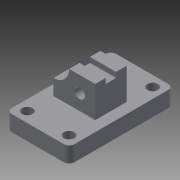
# Autodesk Inventor part: HW 8 Part6
Saved by Autodesk Inventor 2015 (Build 190159000, 159)
## iProperties
Created: 2016-03-08
Part Number: HW 8 Part6
Material: Generic
Document SubType Name: Modeling
Designer: Melissa
Density: 1 g/cm^3
Appearance: Default
Author: Melissa
Autodesk Inventor part; units mm, degrees
ref_plane "YZ Plane" through (0, 0, 0) normal (1, 0, 0) x (0, 1, 0)
ref_plane "XZ Plane" through (0, 0, 0) normal (0, 1, 0) x (-1, 0, 0)
ref_plane "XY Plane" through (0, 0, 0) normal (0, 0, 1) x (1, 0, 0)
sketch "Sketch1" plane through (0, 0, 0) normal (0, 0, 1) x (1, 0, 0)
  line L0 (0, 0) -> (50.8, 0)
  line L1 (50.8, 0) -> (50.8, 38.1)
  line L2 (50.8, 38.1) -> (19.05, 38.1)
  line L3 (0, 19.05) -> (0, 0)
  arc A0 (0, 19.05) -> (19.05, 38.1) centre (0, 38.1) ccw
  circle A1 centre (31.75, 19.05) radius 6.35
  dimension "d0" = 38.1
  dimension "d1" = 50.8
  dimension "d4" = 19.05
  dimension "d5" = 12.7
  dimension "d6" = 19.05
  dimension "d7" = 19.05
  constraints: 8 end point, 2 centre point, 2 horizontal, 2 perpendicular, 2 point on circle
  measures "d0" distance of L0.end L1.end
  measures "d1" distance of L0.start L0.end
  measures "d4" radius of A0
  measures "d5" diameter of A1
  measures "d6" distance from line of L1 A1.centre
  measures "d7" distance from line of L0 A1.centre
extrude "Extrusion1" add sketch "Sketch1" along normal blind 38.1
sketch "Sketch2" plane through (0, 0, 0) normal (0, -1, 0) x (1, 0, 0)
  line L0 (57.15, 82.55) -> (-6.35, 82.55)
  line L1 (-12.7, 76.2) -> (-12.7, -38.1)
  line L2 (-6.35, -44.45) -> (57.15, -44.45)
  line L3 (63.5, -38.1) -> (63.5, 76.2)
  line L4 (0, 0) -> (0, 38.1) projected
  line L5 (0, 0) -> (50.8, 0) projected
  arc A0 (63.5, 76.2) -> (57.15, 82.55) centre (57.15, 76.2) ccw
  arc A1 (-6.35, 82.55) -> (-12.7, 76.2) centre (-6.35, 76.2) ccw
  arc A2 (-12.7, -38.1) -> (-6.35, -44.45) centre (-6.35, -38.1) ccw
  arc A3 (57.15, -44.45) -> (63.5, -38.1) centre (57.15, -38.1) ccw
  circle A4 centre (50.8, -31.75) radius 6.35
  circle A5 centre (0, -31.75) radius 6.35
  circle A6 centre (50.8, 69.85) radius 6.35
  circle A7 centre (0, 69.85) radius 6.35
  point P0 (-12.7, -44.45)
  point P1 (-12.7, 82.55)
  point P2 (63.5, -44.45)
  dimension "d11" = 76.2
  dimension "d12" = 127
  dimension "d13" = 12.7
  dimension "d14" = 44.45
  dimension "d15" = 6.35
  dimension "d16" = 12.7
  dimension "d17" = 12.7
  dimension "d18" = 12.7
  constraints: 8 centre point, 8 end point, 8 point on circle, 8 tangent, 6 point on line, 3 equal radius, 2 parallel, 1 horizontal, 1 perpendicular
  measures "d11" distance of point (-12.7, -44.45) point (63.5, -44.45)
  measures "d12" distance of point (-12.7, 82.55) point (-12.7, -44.45)
  measures "d13" distance between parallel lines of L4 L1
  measures "d14" distance between parallel lines of L2 L5
  measures "d15" radius of A0
  measures "d16" diameter of A4
  measures "d17" distance from line of L2 A4.centre
  measures "d18" distance from line of L3 A4.centre
extrude "Extrusion2" add sketch "Sketch2" along normal blind 19.05
sketch "Sketch3" plane through (19.05, 38.1, 0) normal (0, 1, 0) x (1, 0, 0)
  line L0 (31.75, 0) -> (31.75, -38.1) projected
  line L1 (0, 0) -> (0, -38.1) projected
  line L2 (31.75, -12.7) -> (0, -12.7)
  line L3 (0, -12.7) -> (0, -25.4)
  line L4 (0, -25.4) -> (31.75, -25.4)
  line L5 (31.75, -25.4) -> (31.75, -12.7)
  point P0 (-19.05, 0)
  dimension "d21" = 12.7
  dimension "d22" = 12.7
  constraints: 8 end point, 2 parallel, 2 point on line, 1 horizontal, 1 perpendicular
  measures "d21" distance of L0.start L2.start
  measures "d22" distance of L4.end L2.start
extrude "Extrusion3" cut sketch "Sketch3" against normal blind 6.35
body "Solid1"
